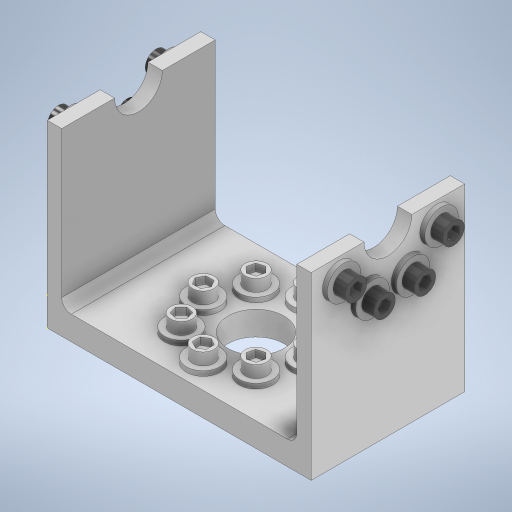
# Autodesk Inventor part: linkzinho_motor
Saved by Autodesk Inventor 2024 (Build 280153000, 153)
## iProperties
Created: 2024-10-14
Part Number: linkzinho_motor
Material: Genérico
Document SubType Name: Modeling
Designer: robof
Density: 1 g/cm^3
Appearance: Padrão
Author: robof
Autodesk Inventor part; units mm, degrees
ref_plane "YZ Plane" through (0, 0, 0) normal (1, 0, 0) x (0, 1, 0)
ref_plane "XZ Plane" through (0, 0, 0) normal (0, 1, 0) x (-1, 0, 0)
ref_plane "XY Plane" through (0, 0, 0) normal (0, 0, 1) x (1, 0, 0)
sketch "Esboço1" plane through (0, 0, 0) normal (0, 1, 0) x (-1, 0, 0)
  line L0 (0, 0) -> (-55, 0)
  line L1 (-55, 0) -> (-55, -32)
  line L2 (-55, -32) -> (0, -32)
  line L3 (0, -32) -> (0, 0)
  dimension "d0" = 55
  dimension "d1" = 32
  constraints: 8 end point, 2 parallel, 1 horizontal, 1 perpendicular
  measures "d0" distance of L2.end L1.end
  measures "d1" distance of L1.end L0.end
extrude "Extrusão1" add sketch "Esboço1" along normal blind 37.5
sketch "Esboço2" plane through (0, 37.5, 0) normal (0, 1, 0) x (1, 0, 0)
  line L0 (55, 32) -> (0, 32) projected
  line L1 (0, 0) -> (3, 0)
  line L2 (3, 0) -> (3, 32)
  line L3 (3, 32) -> (0, 32)
  line L4 (0, 32) -> (0, 0)
  line L5 (55, 0) -> (55, 32) projected
  line L6 (55, 32) -> (52, 32)
  line L7 (52, 32) -> (52, 0)
  line L8 (52, 0) -> (55, 0)
  line L9 (55, 0) -> (55, 32)
  line L10 (3, 32) -> (52, 32)
  line L11 (52, 32) -> (52, 0)
  line L12 (52, 0) -> (3, 0)
  line L13 (3, 0) -> (3, 32)
  dimension "d4" = 3
  dimension "d5" = 3
  constraints: 24 end point, 6 parallel, 3 horizontal, 3 perpendicular, 2 point on line
  measures "d4" distance of L3.end L2.end
  measures "d5" distance of L8.end L7.end
extrude "Extrusão2" cut sketch "Esboço2" against normal blind 32.5 contours L7 L12 L2 L0
sketch "Esboço3" plane through (0, 0, -32) normal (-1, 0, 0) x (0, 0, 1)
  line L0 (32, 37.5) -> (0, 37.5) projected
  circle A0 centre (16, 37.5) radius 4.975
  point P0 (32, 0)
  point P1 (11.025, 37.5)
  point P2 (20.975, 37.5)
  dimension "d8" = 9.95
  constraints: 1 centre point, 1 midpoint
  measures "d8" diameter of A0
extrude "Extrusão3" cut sketch "Esboço3" against normal blind 100 contours A0 L0 picked at (17.6101, 37.1031)
sketch "Esboço4" plane through (0, 0, -32) normal (-1, 0, 0) x (0, 0, 1)
  arc A0 (11.025, 37.5) -> (20.975, 37.5) centre (16, 37.5) ccw projected
  line L0 (16, 37.5) -> (27, 37.5) construction
  line L1 (16, 37.5) -> (26.1627, 33.2905)
  line L2 (16, 37.5) -> (27, 37.5) construction
  line L3 (16, 37.5) -> (20.2095, 27.3373)
  line L4 (16, 37.5) -> (27, 37.5) construction
  line L5 (16, 37.5) -> (5.8373, 33.2905)
  line L6 (16, 37.5) -> (11.7905, 27.3373)
  circle A1 centre (5.8373, 33.2905) radius 3.5
  circle A2 centre (11.7905, 27.3373) radius 3.5
  circle A3 centre (20.2095, 27.3373) radius 3.5
  circle A4 centre (26.1627, 33.2905) radius 3.5
  point P0 (32, 0)
  dimension "d18" = 7
  dimension "d19" = 7
  dimension "d20" = 7
  dimension "d21" = 7
  constraints: 14 end point, 4 centre point, 4 coincident, 3 horizontal, 2 equal length
  measures "d18" diameter of A1
  measures "d19" diameter of A2
  measures "d20" diameter of A3
  measures "d21" diameter of A4
extrude "Extrusão4" add sketch "Esboço4" along normal blind 1 contours A1 | A2 | A3 | A4
sketch "Esboço5" plane through (-1, 33.2905, -26.1627) normal (-1, 0, 0) x (0, 0, 1)
  circle A0 centre (0, 0) radius 3.5 projected
  circle A1 centre (0, 0) radius 2.25
  circle A2 centre (5.9532, -5.9532) radius 3.5 projected
  circle A3 centre (5.9532, -5.9532) radius 2.25
  circle A4 centre (14.3722, -5.9532) radius 3.5 projected
  circle A5 centre (14.3722, -5.9532) radius 2.25
  circle A6 centre (20.3253, 0) radius 3.5 projected
  circle A7 centre (20.3253, 0) radius 2.25
  point P0 (26.1627, -33.2905)
  dimension "d24" = 4.5
  dimension "d25" = 4.5
  dimension "d26" = 4.5
  constraints: 4 centre point, 4 coincident
  measures "d24" diameter of A1
  measures "d25" diameter of A3
  measures "d26" diameter of A5
extrude "Extrusão5" add sketch "Esboço5" along normal blind 2.5 contours A1 | A3 | A5 | A7
sketch "Esboço6" plane through (-3.5, 33.2905, -26.1627) normal (-1, 0, 0) x (0, 0, 1)
  line L0 (-0.0054, -1.3725) -> (-1.1913, -0.6816)
  line L1 (-1.1913, -0.6816) -> (-1.1859, 0.6909)
  line L2 (-1.1859, 0.6909) -> (0.0054, 1.3725)
  line L3 (0.0054, 1.3725) -> (1.1913, 0.6816)
  line L4 (1.1913, 0.6816) -> (1.1859, -0.6909)
  line L5 (1.1859, -0.6909) -> (-0.0054, -1.3725)
  arc A0 (5.1877, 4.2095) -> (15.1377, 4.2095) centre (10.1627, 4.2095) ccw projected
  circle A1 centre (10.1627, 4.2095) radius 4.975
  line L6 (6.9199, -6.9275) -> (5.5927, -7.2775)
  line L7 (5.5927, -7.2775) -> (4.626, -6.3032)
  line L8 (4.626, -6.3032) -> (4.9864, -4.9788)
  line L9 (4.9864, -4.9788) -> (6.3136, -4.6288)
  line L10 (6.3136, -4.6288) -> (7.2803, -5.6031)
  line L11 (7.2803, -5.6031) -> (6.9199, -6.9275)
  line L12 (15.7447, -5.9585) -> (15.0538, -7.1445)
  line L13 (15.0538, -7.1445) -> (13.6813, -7.1391)
  line L14 (13.6813, -7.1391) -> (12.9997, -5.9478)
  line L15 (12.9997, -5.9478) -> (13.6906, -4.7618)
  line L16 (13.6906, -4.7618) -> (15.0631, -4.7672)
  line L17 (15.0631, -4.7672) -> (15.7447, -5.9585)
  line L18 (21.2997, 0.9667) -> (21.6497, -0.3604)
  line L19 (21.6497, -0.3604) -> (20.6754, -1.3271)
  line L20 (20.6754, -1.3271) -> (19.351, -0.9667)
  line L21 (19.351, -0.9667) -> (19.001, 0.3604)
  line L22 (19.001, 0.3604) -> (19.9753, 1.3271)
  line L23 (19.9753, 1.3271) -> (21.2997, 0.9667)
  line L24 (20.3307, 9.7915) -> (21.5167, 9.1006)
  line L25 (21.5167, 9.1006) -> (21.5113, 7.7281)
  line L26 (21.5113, 7.7281) -> (20.32, 7.0465)
  line L27 (20.32, 7.0465) -> (19.134, 7.7374)
  line L28 (19.134, 7.7374) -> (19.1394, 9.1099)
  line L29 (19.1394, 9.1099) -> (20.3307, 9.7915)
  line L30 (13.4055, 15.3465) -> (14.7326, 15.6965)
  line L31 (14.7326, 15.6965) -> (15.6993, 14.7222)
  line L32 (15.6993, 14.7222) -> (15.3389, 13.3979)
  line L33 (15.3389, 13.3979) -> (14.0118, 13.0478)
  line L34 (14.0118, 13.0478) -> (13.0451, 14.0222)
  line L35 (13.0451, 14.0222) -> (13.4055, 15.3465)
  line L36 (4.5806, 14.3776) -> (5.2716, 15.5635)
  line L37 (5.2716, 15.5635) -> (6.6441, 15.5581)
  line L38 (6.6441, 15.5581) -> (7.3257, 14.3668)
  line L39 (7.3257, 14.3668) -> (6.6348, 13.1809)
  line L40 (6.6348, 13.1809) -> (5.2622, 13.1863)
  line L41 (5.2622, 13.1863) -> (4.5806, 14.3776)
  line L42 (-0.9743, 7.4523) -> (-1.3244, 8.7795)
  line L43 (-1.3244, 8.7795) -> (-0.35, 9.7462)
  line L44 (-0.35, 9.7462) -> (0.9743, 9.3857)
  line L45 (0.9743, 9.3857) -> (1.3244, 8.0586)
  line L46 (1.3244, 8.0586) -> (0.35, 7.0919)
  line L47 (0.35, 7.0919) -> (-0.9743, 7.4523)
  point P0 (26.1627, -33.2905)
  point P1 (0, 0)
  point P2 (5.9532, -5.9532)
  point P3 (14.3722, -5.9532)
  point P4 (20.3253, 0)
  point P5 (20.3253, 8.419)
  point P6 (14.3722, 14.3722)
  point P7 (5.9532, 14.3722)
  point P8 (0, 8.419)
  dimension "d31" = 360
  constraints: 96 end point, 1 centre point, 1 coincident, 118 other
extrude "Extrusão6" cut sketch "Esboço6" against normal blind 1.5 contours L0 L1 L2 L3 L4 L5 | L6 L7 L8 L9 L10 L11 | L12 L13 L14 L15 L16 L17 | L18 L19 L20 L21 L22 L23
sketch "Esboço7" plane through (55, 0, 0) normal (1, 0, 0) x (0, 0, -1)
  circle A0 centre (26.1627, 33.2905) radius 3.5 projected
  circle A1 centre (26.1627, 33.2905) radius 3.5
  circle A2 centre (20.2095, 27.3373) radius 2.25 projected
  circle A3 centre (20.2095, 27.3373) radius 3.5
  circle A4 centre (11.7905, 27.3373) radius 3.5 projected
  circle A5 centre (11.7905, 27.3373) radius 3.5
  circle A6 centre (5.8373, 33.2905) radius 3.5 projected
  circle A7 centre (5.8373, 33.2905) radius 3.5
  point P0 (0, 0)
  dimension "d35" = 7
  constraints: 4 centre point, 4 coincident
  measures "d35" diameter of A3
extrude "Extrusão7" add sketch "Esboço7" along normal blind 1 contours A0 | A2 | A3 | A4 | A6
sketch "Esboço8" plane through (56, 33.2905, -5.8373) normal (1, 0, 0) x (0, 0, -1)
  circle A0 centre (0, 0) radius 2.25
  circle A1 centre (5.9532, -5.9532) radius 2.25 projected
  circle A2 centre (5.9532, -5.9532) radius 2.25
  circle A3 centre (14.3722, -5.9532) radius 2.25 projected
  circle A4 centre (14.3722, -5.9532) radius 2.25
  circle A5 centre (20.3253, 0) radius 2.25 projected
  circle A6 centre (20.3253, 0) radius 2.25
  point P0 (-5.8373, -33.2905)
  constraints: 4 centre point, 3 coincident
extrude "Extrusão8" add sketch "Esboço8" along normal blind 2.5
sketch "Esboço9" plane through (58.5, 33.2905, -5.8373) normal (1, 0, 0) x (0, 0, -1)
  line L0 (-1.3244, -0.3604) -> (-0.35, -1.3271) projected
  line L1 (-0.35, -1.3271) -> (-1.3244, -0.3604)
  line L2 (-1.3244, -0.3604) -> (-0.9743, 0.9667)
  line L3 (-0.9743, 0.9667) -> (0.35, 1.3271)
  line L4 (0.35, 1.3271) -> (1.3244, 0.3604)
  line L5 (1.3244, 0.3604) -> (0.9743, -0.9667)
  line L6 (0.9743, -0.9667) -> (-0.35, -1.3271)
  arc A0 (5.1877, 4.2095) -> (15.1377, 4.2095) centre (10.1627, 4.2095) ccw projected
  circle A1 centre (10.1627, 4.2095) radius 4.975
  line L7 (6.6441, -7.1391) -> (5.2716, -7.1445)
  line L8 (5.2716, -7.1445) -> (4.5806, -5.9585)
  line L9 (4.5806, -5.9585) -> (5.2622, -4.7672)
  line L10 (5.2622, -4.7672) -> (6.6348, -4.7618)
  line L11 (6.6348, -4.7618) -> (7.3257, -5.9478)
  line L12 (7.3257, -5.9478) -> (6.6441, -7.1391)
  line L13 (15.6993, -6.3032) -> (14.7326, -7.2775)
  line L14 (14.7326, -7.2775) -> (13.4055, -6.9275)
  line L15 (13.4055, -6.9275) -> (13.0451, -5.6031)
  line L16 (13.0451, -5.6031) -> (14.0118, -4.6288)
  line L17 (14.0118, -4.6288) -> (15.3389, -4.9788)
  line L18 (15.3389, -4.9788) -> (15.6993, -6.3032)
  line L19 (21.5113, 0.6909) -> (21.5167, -0.6816)
  line L20 (21.5167, -0.6816) -> (20.3307, -1.3725)
  line L21 (20.3307, -1.3725) -> (19.1394, -0.6909)
  line L22 (19.1394, -0.6909) -> (19.134, 0.6816)
  line L23 (19.134, 0.6816) -> (20.32, 1.3725)
  line L24 (20.32, 1.3725) -> (21.5113, 0.6909)
  line L25 (20.6754, 9.7462) -> (21.6497, 8.7795)
  line L26 (21.6497, 8.7795) -> (21.2997, 7.4523)
  line L27 (21.2997, 7.4523) -> (19.9753, 7.0919)
  line L28 (19.9753, 7.0919) -> (19.001, 8.0586)
  line L29 (19.001, 8.0586) -> (19.351, 9.3857)
  line L30 (19.351, 9.3857) -> (20.6754, 9.7462)
  line L31 (13.6813, 15.5581) -> (15.0538, 15.5635)
  line L32 (15.0538, 15.5635) -> (15.7447, 14.3776)
  line L33 (15.7447, 14.3776) -> (15.0631, 13.1863)
  line L34 (15.0631, 13.1863) -> (13.6906, 13.1809)
  line L35 (13.6906, 13.1809) -> (12.9997, 14.3668)
  line L36 (12.9997, 14.3668) -> (13.6813, 15.5581)
  line L37 (4.626, 14.7222) -> (5.5927, 15.6965)
  line L38 (5.5927, 15.6965) -> (6.9199, 15.3465)
  line L39 (6.9199, 15.3465) -> (7.2803, 14.0222)
  line L40 (7.2803, 14.0222) -> (6.3136, 13.0478)
  line L41 (6.3136, 13.0478) -> (4.9864, 13.3979)
  line L42 (4.9864, 13.3979) -> (4.626, 14.7222)
  line L43 (-1.1859, 7.7281) -> (-1.1913, 9.1006)
  line L44 (-1.1913, 9.1006) -> (-0.0054, 9.7915)
  line L45 (-0.0054, 9.7915) -> (1.1859, 9.1099)
  line L46 (1.1859, 9.1099) -> (1.1913, 7.7374)
  line L47 (1.1913, 7.7374) -> (0.0054, 7.0465)
  line L48 (0.0054, 7.0465) -> (-1.1859, 7.7281)
  point P0 (-5.8373, -33.2905)
  point P1 (0, 0)
  point P2 (5.9532, -5.9532)
  point P3 (14.3722, -5.9532)
  point P4 (20.3253, 0)
  point P5 (20.3253, 8.419)
  point P6 (14.3722, 14.3722)
  point P7 (5.9532, 14.3722)
  point P8 (0, 8.419)
  dimension "d42" = 360
  constraints: 96 end point, 1 coincident, 1 horizontal alignment, 120 other
extrude "Extrusão9" cut sketch "Esboço9" against normal blind 1.5 contours L2 L3 L4 L5 L6 L0 | L7 L8 L9 L10 L11 L12 | L13 L14 L15 L16 L17 L18 | L19 L20 L21 L22 L23 L24
fillet "Arredondamento1" radius 2 2 edges at (3, 5, -16) (52, 5, -16)
sketch "Esboço10" plane through (0, 0, 0) normal (0, 0, 1) x (1, 0, 0)
  point P0 (0, 0)
sketch "Esboço11" plane through (0, 5, 0) normal (0, 1, 0) x (1, 0, 0)
  line L0 (0, 0) -> (55, 0) projected
  line L1 (55, 32) -> (0, 32) projected
  circle A0 centre (27.5, 16) radius 5.85
  line L2 (27.5, 16) -> (38.5, 16)
  line L3 (27.5, 16) -> (35.2782, 8.2218)
  line L4 (27.5, 16) -> (38.5, 16) construction
  line L5 (27.5, 16) -> (27.5, 5)
  line L6 (27.5, 16) -> (27.5, 27)
  line L7 (27.5, 16) -> (35.2782, 23.7782)
  line L8 (27.5, 16) -> (16.5, 16)
  line L9 (27.5, 16) -> (19.7218, 23.7782)
  circle A1 centre (27.5, 27) radius 3.5
  circle A2 centre (35.2782, 23.7782) radius 3.5
  circle A3 centre (38.5, 16) radius 3.5
  circle A4 centre (35.2782, 8.2218) radius 3.5
  circle A5 centre (27.5, 5) radius 3.5
  circle A6 centre (16.5, 16) radius 3.5
  circle A7 centre (20, 23.5) radius 3.5
  line L10 (27.5, 16) -> (20, 7.9533)
  circle A8 centre (20, 7.9533) radius 3.5
  dimension "d47" = 11.7
  dimension "d48" = 11
  dimension "d49" = 11
  dimension "d50" = 45
  dimension "d51" = 11
  dimension "d52" = 11
  dimension "d53" = 11
  dimension "d54" = 7
  dimension "d55" = 7
  dimension "d56" = 7
  dimension "d57" = 7
  dimension "d58" = 7
  dimension "d59" = 7
  dimension "d60" = 7
  dimension "d61" = 11
  dimension "d62" = 7
  constraints: 18 end point, 9 centre point, 7 coincident, 3 horizontal, 2 vertical, 1 equal length, 1 perpendicular, 1 point on line
  measures "d47" diameter of A0
  measures "d48" distance of L2.start L2.end
  measures "d49" distance of L2.start L3.end
  measures "d50" angle of L3 L4
  measures "d51" distance of L2.start L5.end
  measures "d52" distance of L2.start L6.end
  measures "d53" distance of L2.start L8.end
  measures "d54" diameter of A1
  measures "d55" diameter of A2
  measures "d56" diameter of A3
  measures "d57" diameter of A4
  measures "d58" diameter of A5
  measures "d59" diameter of A6
  measures "d60" diameter of A7
  measures "d61" distance of L2.start L10.end
  measures "d62" diameter of A8
extrude "Extrusão10" add sketch "Esboço11" along normal blind 1
sketch "Esboço12" plane through (27.5, 6, -16) normal (0, 1, 0) x (1, 0, 0)
  point P0 (-27.5, -16)
sketch "Esboço13" plane through (27.5, 6, -16) normal (0, 1, 0) x (1, 0, 0)
  circle A0 centre (0, 0) radius 5.85 projected
  circle A1 centre (0, 0) radius 5.85
  point P0 (-27.5, -16)
  constraints: 1 centre point, 1 coincident
extrude "Extrusão11" cut sketch "Esboço13" against normal blind 10
sketch "Esboço14" plane through (27.5, 6, -27) normal (0, 1, 0) x (1, 0, 0)
  circle A0 centre (0, 0) radius 2.25
  circle A1 centre (-7.5, -19.0467) radius 3.5 projected
  circle A2 centre (-7.5, -19.0467) radius 3.5
  point P0 (-27.5, -27)
  dimension "d67" = 4.5
  constraints: 2 centre point, 1 coincident
  measures "d67" diameter of A0
extrude "Extrusão12" cut sketch "Esboço14" against normal blind 1 contours A1
sketch "Esboço15" plane through (35.2782, 6, -23.7782) normal (0, 1, 0) x (1, 0, 0)
  circle A0 centre (-7.7782, -7.7782) radius 5.85 projected
  line L0 (-7.7782, -7.7782) -> (3.4481, -7.7782) construction
  circle A1 centre (0, 0) radius 3.5 projected
  circle A2 centre (0, 0) radius 3.5
  circle A3 centre (-15.5563, -15.5563) radius 3.5
  circle A4 centre (0, 0) radius 2.25
  circle A5 centre (-15.2782, -0.2782) radius 3.5 projected
  circle A6 centre (-15.2782, -0.2782) radius 3.5
  point P0 (-35.2782, -23.7782)
  dimension "d71" = 4.5
  constraints: 4 centre point, 3 coincident, 2 end point, 1 horizontal
  measures "d71" diameter of A4
extrude "Extrusão13" cut sketch "Esboço15" against normal blind 1 contours A5
sketch "Esboço16" plane through (0, 5, 0) normal (0, 1, 0) x (1, 0, 0)
  circle A0 centre (27.5, 16) radius 5.85 projected
  line L0 (27.5, 16) -> (34.8396, 8.6604)
  line L1 (27.5, 16) -> (37.8798, 16) construction
  line L2 (27.5, 16) -> (18.9904, 16)
  circle A1 centre (35.2782, 23.7782) radius 3.5 projected
  circle A2 centre (35.2782, 23.7782) radius 3.5
  circle A3 centre (19.7218, 8.2218) radius 3.5
  circle A4 centre (19.7218, 23.7782) radius 3.5
  point P0 (0, 0)
  dimension "d74" = 45
  constraints: 6 end point, 3 centre point, 2 horizontal, 2 symmetric about line, 1 coincident, 1 equal length, 2 other
  measures "d74" angle of L0 L1
extrude "Extrusão14" add sketch "Esboço16" along normal blind 1 contours A3 | A4
sketch "Esboço17" plane through (27.5, 6, -27) normal (0, 1, 0) x (1, 0, 0)
  circle A0 centre (0, 0) radius 3.5 projected
  circle A1 centre (0, 0) radius 2.25
  circle A2 centre (0, -11) radius 5.85 projected
  circle A3 centre (0, -11) radius 5.85
  circle A4 centre (-7.7782, -3.2218) radius 2.25
  circle A5 centre (-11, -11) radius 2.25
  circle A6 centre (-7.7782, -18.7782) radius 2.25
  circle A7 centre (0, -22) radius 2.25
  circle A8 centre (7.7782, -18.7782) radius 2.25
  circle A9 centre (11, -11) radius 2.25
  circle A10 centre (7.7782, -3.2218) radius 2.25
  point P0 (-27.5, -27)
  dimension "d77" = 4.5
  dimension "d80" = 360
  constraints: 9 centre point, 2 coincident, 17 other
  measures "d77" diameter of A1
extrude "Extrusão15" add sketch "Esboço17" along normal blind 2.5 contours A1 | A4 | A5 | A6 | A7 | A8 | A9 | A10
sketch "Esboço18" plane through (27.5, 8.5, -27) normal (0, 1, 0) x (1, 0, 0)
  line L0 (0.0376, -1.667) -> (-1.4248, -0.8661)
  line L1 (-1.4248, -0.8661) -> (-1.4625, 0.8009)
  line L2 (-1.4625, 0.8009) -> (-0.0376, 1.667)
  line L3 (-0.0376, 1.667) -> (1.4248, 0.8661)
  line L4 (1.4248, 0.8661) -> (1.4625, -0.8009)
  line L5 (1.4625, -0.8009) -> (0.0376, -1.667)
  circle A0 centre (0, -11) radius 5.85 projected
  circle A1 centre (0, -11) radius 5.85
  line L6 (-6.5728, -4.374) -> (-8.1733, -4.8418)
  line L7 (-8.1733, -4.8418) -> (-9.3786, -3.6896)
  line L8 (-9.3786, -3.6896) -> (-8.9835, -2.0697)
  line L9 (-8.9835, -2.0697) -> (-7.3831, -1.6019)
  line L10 (-7.3831, -1.6019) -> (-6.1777, -2.754)
  line L11 (-6.1777, -2.754) -> (-6.5728, -4.374)
  line L12 (-9.333, -10.9624) -> (-10.1339, -12.4248)
  line L13 (-10.1339, -12.4248) -> (-11.8009, -12.4625)
  line L14 (-11.8009, -12.4625) -> (-12.667, -11.0376)
  line L15 (-12.667, -11.0376) -> (-11.8661, -9.5752)
  line L16 (-11.8661, -9.5752) -> (-10.1991, -9.5375)
  line L17 (-10.1991, -9.5375) -> (-9.333, -10.9624)
  line L18 (-6.626, -17.5728) -> (-6.1582, -19.1733)
  line L19 (-6.1582, -19.1733) -> (-7.3104, -20.3786)
  line L20 (-7.3104, -20.3786) -> (-8.9303, -19.9835)
  line L21 (-8.9303, -19.9835) -> (-9.3981, -18.3831)
  line L22 (-9.3981, -18.3831) -> (-8.246, -17.1777)
  line L23 (-8.246, -17.1777) -> (-6.626, -17.5728)
  line L24 (-0.0376, -20.333) -> (1.4248, -21.1339)
  line L25 (1.4248, -21.1339) -> (1.4625, -22.8009)
  line L26 (1.4625, -22.8009) -> (0.0376, -23.667)
  line L27 (0.0376, -23.667) -> (-1.4248, -22.8661)
  line L28 (-1.4248, -22.8661) -> (-1.4625, -21.1991)
  line L29 (-1.4625, -21.1991) -> (-0.0376, -20.333)
  line L30 (6.5728, -17.626) -> (8.1733, -17.1582)
  line L31 (8.1733, -17.1582) -> (9.3786, -18.3104)
  line L32 (9.3786, -18.3104) -> (8.9835, -19.9303)
  line L33 (8.9835, -19.9303) -> (7.3831, -20.3981)
  line L34 (7.3831, -20.3981) -> (6.1777, -19.246)
  line L35 (6.1777, -19.246) -> (6.5728, -17.626)
  line L36 (9.333, -11.0376) -> (10.1339, -9.5752)
  line L37 (10.1339, -9.5752) -> (11.8009, -9.5375)
  line L38 (11.8009, -9.5375) -> (12.667, -10.9624)
  line L39 (12.667, -10.9624) -> (11.8661, -12.4248)
  line L40 (11.8661, -12.4248) -> (10.1991, -12.4625)
  line L41 (10.1991, -12.4625) -> (9.333, -11.0376)
  line L42 (6.626, -4.4272) -> (6.1582, -2.8267)
  line L43 (6.1582, -2.8267) -> (7.3104, -1.6214)
  line L44 (7.3104, -1.6214) -> (8.9303, -2.0165)
  line L45 (8.9303, -2.0165) -> (9.3981, -3.6169)
  line L46 (9.3981, -3.6169) -> (8.246, -4.8223)
  line L47 (8.246, -4.8223) -> (6.626, -4.4272)
  point P0 (-27.5, -27)
  point P1 (0, 0)
  point P2 (-7.7782, -3.2218)
  point P3 (-11, -11)
  point P4 (-7.7782, -18.7782)
  point P5 (0, -22)
  point P6 (7.7782, -18.7782)
  point P7 (11, -11)
  point P8 (7.7782, -3.2218)
  dimension "d86" = 360
  constraints: 96 end point, 1 centre point, 1 coincident, 118 other
extrude "Extrusão16" cut sketch "Esboço18" against normal blind 1.5 contours L0 L1 L2 L3 L4 L5 | L6 L7 L8 L9 L10 L11 | L12 L13 L14 L15 L16 L17 | L18 L19 L20 L21 L22 L23 | L24 L25 L26 L27 L28 L29 | L30 L31 L32 L33 L34 L35 | L36 L37 L38 L39 L40 L41 | L42 L43 L44 L45 L46 L47
